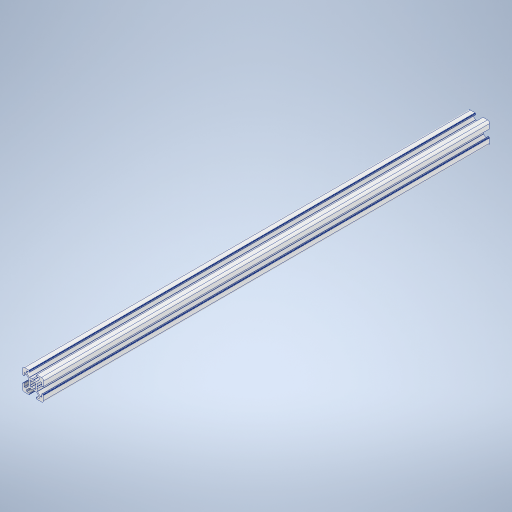
# Autodesk Inventor part: AluminiumTSlotProfil20x20x420
Saved by Autodesk Inventor 2024 (Build 280153000, 153)
## iProperties
Created: 2023-12-26
Part Number: AluminiumTSlotProfil20x20x420
Material: Generisch
Document SubType Name: Modeling
Designer: denni
Density: 1 g/cm^3
Appearance: Aluminium - flach
Author: denni
Autodesk Inventor part; units mm, degrees
ref_plane "YZ Plane" through (0, 0, 0) normal (1, 0, 0) x (0, 1, 0)
ref_plane "XZ Plane" through (0, 0, 0) normal (0, 1, 0) x (-1, 0, 0)
ref_plane "XY Plane" through (0, 0, 0) normal (0, 0, 1) x (1, 0, 0)
sketch "Skizze1" plane through (0, 0, 0) normal (0, 0, 1) x (1, 0, 0)
  line L0 (0, 2.65) -> (0, 0) construction
  line L1 (0, 2.65) -> (0, 3.81)
  line L2 (0, 0) -> (10, 10) construction
  line L3 (0.875, 4.31) -> (4.31, 4.31)
  line L4 (0, 3.81) -> (0.875, 4.31)
  arc A0 (1.3347, 2.2893) -> (0, 2.65) centre (0, 0) ccw
  line L5 (2.4749, 2.4749) -> (1.9976, 2.9522)
  line L6 (1.9976, 2.9522) -> (1.3347, 2.2893)
  line L7 (10, 10) -> (3, 10)
  line L8 (3, 10) -> (3, 8.4)
  line L9 (3, 8.4) -> (7.3393, 8.4)
  line L10 (7.3393, 8.4) -> (3.2493, 4.31)
  line L11 (4.31, 4.31) -> (10, 10)
  line L12 (6, 8.4) -> (6, 7.0607)
  arc A1 (9.4142, 9.4142) -> (8, 10) centre (8, 8) ccw
  line L13 (4.31, 4.31) -> (2.4749, 2.4749)
  line L14 (3, 10) -> (3.6, 10)
  line L15 (3.6, 10) -> (3.6, 9.4)
  line L16 (3.6, 9.4) -> (3, 9.4)
  line L17 (3, 9.4) -> (3, 10)
  arc A2 (0, 3.8176) -> (0.0248, 3.8242) centre (0, 3.8676) ccw
  line L18 (0, 3.81) -> (0, 3.8176)
  dimension "d0" = 45
  dimension "d1" = 8.62
  dimension "d2" = 1.75
  dimension "d3" = 0.5
  dimension "d4" = 2.65
  dimension "d5" = 3.5
  dimension "d6" = 1.35
  dimension "d7" = 7
  dimension "d8" = 20
  dimension "d9" = 1.6
  dimension "d10" = 1.5
  dimension "d11" = 4
  dimension "d12" = 2
  dimension "d13" = 1
  dimension "d18" = 0.05
  constraints: 38 end point, 9 point on line, 6 perpendicular, 6 point on circle, 4 vertical, 3 centre point, 3 horizontal, 3 parallel, 2 coincident, 2 tangent, 1 collinear, 1 line through centre
  measures "d0" angle of L2 L0
  measures "d1" diameter of L3.end L0
  measures "d2" diameter of L3.start L0
  measures "d3" distance from line of L1.end L3
  measures "d4" radius of A0
  measures "d5" distance from line of point (0, 0) L5
  measures "d6" diameter of L6 L2
  measures "d7" distance of L2.end L7.end
  measures "d8" diameter of L2.end L0
  measures "d9" distance of L7.end L8.end
  measures "d10" diameter of L10 L2
  measures "d11" distance from line of L2.end L12
  measures "d12" radius of A1
  measures "d13" distance between parallel lines of L9 L16
  measures "d18" radius of A2
extrude "Extrusion1" add sketch "Skizze1" along normal blind 420 contours L1 L4 L3 L13 L5 L6 A0 | L18 A2 L4 | L10 L9 L8 L16 L15 L7 A1 L11 L3 | L12 L9 L10
fillet "Rundung1" radius 0.3 5 edges at (3, 8.4, 210) (3, 9.4, 210) (6, 8.4, 210) (6, 7.0607, 210) (3.2493, 4.31, 210)
fillet "Rundung2" radius 0.1 5 edges at (3.6, 9.4, 210) (3.6, 10, 210) (0.875, 4.31, 210) (1.9976, 2.9522, 210) (1.3347, 2.2893, 210)
mirror "Spiegeln1" about plane through (2.4749, 2.4749, 0) normal (0.7071068, -0.7071068, 0) of "Extrusion1", "Rundung1", "Rundung2"
pattern_circular "Runde Anordnung1" count 4 over 360 about axis through (0, 0, -10) along (0, 0, 1) of "Extrusion1", "Rundung1", "Rundung2", "Spiegeln1"
